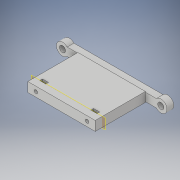
# Autodesk Inventor part: license_mount
Saved by Autodesk Inventor 2019 (Build 230136000, 136)
## iProperties
Created: 2019-09-05
Part Number: license_mount
Material: Generic
Document SubType Name: Modeling
Designer: steve
Density: 1 g/cm^3
Appearance: Default
Author: steve
Autodesk Inventor part; units mm, degrees
ref_plane "YZ Plane" through (0, 0, 0) normal (1, 0, 0) x (0, 1, 0)
ref_plane "XZ Plane" through (0, 0, 0) normal (0, 1, 0) x (-1, 0, 0)
ref_plane "XY Plane" through (0, 0, 0) normal (0, 0, 1) x (1, 0, 0)
sketch "Sketch1" plane through (0, 0, 0) normal (0, 0, 1) x (1, 0, 0)
  circle A0 centre (100.5809, -7) radius 2.5
  circle A1 centre (25.1452, -7) radius 2.5
  line L0 (0, 0) -> (125.7261, 0)
  line L1 (13.1452, 0) -> (112.5809, 0)
  line L2 (112.5809, 0) -> (112.5809, -14)
  line L3 (112.5809, -14) -> (13.1452, -14)
  line L4 (13.1452, -14) -> (13.1452, 0)
  dimension "d0" = 5
  dimension "d1" = 100.5809
  dimension "d2" = 125.7261
  dimension "d3" = 25.1452
  dimension "d4" = 7
  dimension "d5" = 7
  dimension "d8" = 12
  dimension "d9" = 12
  dimension "d10" = 7
  dimension "d23" = 99.4357
  constraints: 10 end point, 2 centre point, 2 horizontal, 2 parallel, 1 coincident, 1 equal radius, 1 perpendicular, 1 point on line
  measures "d0" diameter of A0
  measures "d1" horizontal distance of L0.start A0.centre
  measures "d2" distance of L0.start L0.end
  measures "d3" horizontal distance of L0.start A1.centre
  measures "d4" distance from line of L0 A0.centre
  measures "d5" distance from line of L0 A1.centre
  measures "d8" distance from line of A0.centre L2
  measures "d9" distance from line of A1.centre L4
  measures "d10" distance from line of L3 A0.centre
  measures "d23" distance between parallel lines of L2 L4
extrude "Extrusion1" add sketch "Sketch1" along normal blind 74
ref_plane "Work Plane1" through (0, 0, 64) normal (0, 0, 1) x (1, 0, 0)
sketch "Sketch2" plane through (0, 0, 64) normal (0, 0, 1) x (1, 0, 0)
  circle A0 centre (25.1452, -7) radius 2.5 projected
  circle A1 centre (100.5809, -7) radius 2.5 projected
  line L0 (25.1452, -12.1962) -> (20.6452, -9.5981)
  line L1 (20.6452, -9.5981) -> (20.6452, 0)
  line L2 (29.6452, 0) -> (29.6452, -9.5981)
  line L3 (29.6452, -9.5981) -> (25.1452, -12.1962)
  line L4 (100.5809, -12.1962) -> (96.0809, -9.5981)
  line L5 (96.0809, -9.5981) -> (96.0809, 0)
  line L6 (105.0809, 0) -> (105.0809, -9.5981)
  line L7 (105.0809, -9.5981) -> (100.5809, -12.1962)
  line L8 (13.1452, 0) -> (112.5809, 0) projected
  line L9 (20.6452, 0) -> (29.6452, 0)
  line L10 (96.0809, 0) -> (105.0809, 0)
  point P0 (0, 0)
  dimension "d27" = 9
  dimension "d28" = 9
  constraints: 20 end point, 4 point on line, 2 coincident, 2 collinear, 2 vertical, 12 other
  measures "d27" distance between parallel lines of L2 L1
  measures "d28" distance between parallel lines of L6 L5
extrude "Extrusion2" cut sketch "Sketch2" against normal blind 4 contours A0 | L8 L6 L7 L4 L5 | L0 L1 L8 L2 L3
sketch "Sketch3" plane through (0, 0, 0) normal (0, 0, -1) x (-1, 0, 0)
  circle A0 centre (-135.3631, -7) radius 4.5
  circle A1 centre (9.6369, -7) radius 4.5
  arc A2 (-128.6549, -1) -> (-128.6549, -13) centre (-135.3631, -7) ccw
  arc A3 (2.9287, -13) -> (2.9287, -1) centre (9.6369, -7) ccw
  line L0 (-134.0226, -7) -> (-135.886, -7) construction
  line L1 (-135.886, -7) -> (31.817, -7) construction
  line L2 (-112.5809, -14) -> (-13.1452, -14) construction
  line L3 (-13.1452, 0) -> (-112.5809, 0) construction
  line L4 (-128.6549, -1) -> (2.9287, -1)
  line L5 (2.9287, -13) -> (-128.6549, -13)
  circle A4 centre (-100.5809, -7) radius 2.5 projected
  circle A5 centre (-25.1452, -7) radius 2.5 projected
  point P0 (0, 0)
  dimension "d32" = 145
  dimension "d33" = 9
  dimension "d34" = 18
  dimension "d35" = 14
  dimension "d36" = 7
  dimension "d40" = 12
  dimension "d42" = 75.4357
  dimension "d43" = 34.7822
  constraints: 8 end point, 4 centre point, 4 point on circle, 3 point on line, 2 coincident, 2 equal radius, 2 horizontal, 2 parallel
  measures "d32" distance of A0.centre A1.centre
  measures "d33" diameter of A0
  measures "d34" diameter of A2
  measures "d35" distance between parallel lines of L2 L3
  measures "d36" distance from line of point (0, 0) L1
  measures "d40" distance between parallel lines of L5 L4
  measures "d42" distance of A5.centre A4.centre
  measures "d43" distance of A4.centre A0.centre
extrude "Extrusion3" add sketch "Sketch3" along normal blind 10
equation "\"d1\" = 0.8 * d2"
equation "\"d3\" = 0.2 * d2"
equation "\"d5\" = d4"
equation "\"d9\" = d8"
equation "\"d28\" = d27"
equation "\"d36\" = 0.5 * d35"
equation "\"d43\" = -0.5 * d42 + 0.5 * d32"
body "Solid1"
